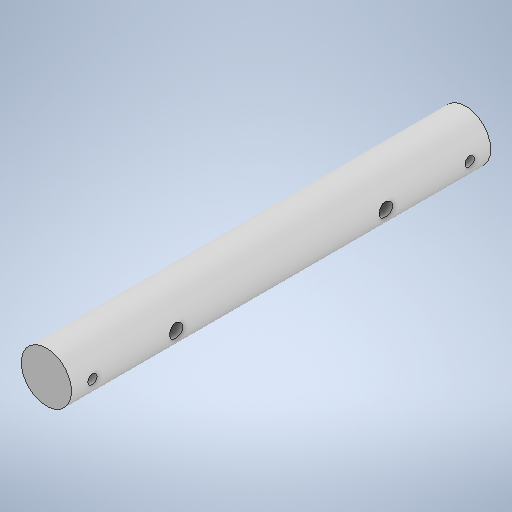
# Autodesk Inventor part: xx_jiku_kakudo
Saved by Autodesk Inventor 2025.1 (Build 291241000, 241)
## iProperties
Created: 2024-12-04
Part Number: xx_jiku_kakudo
Material: 一般
Document SubType Name: Modeling
Designer: yuki0520
Density: 1 g/cm^3
Appearance: 既定
Author: yuki0520
Autodesk Inventor part; units mm, degrees
ref_plane "YZ Plane" through (0, 0, 0) normal (1, 0, 0) x (0, 1, 0)
ref_plane "XZ Plane" through (0, 0, 0) normal (0, 1, 0) x (-1, 0, 0)
ref_plane "XY Plane" through (0, 0, 0) normal (0, 0, 1) x (1, 0, 0)
sketch "スケッチ1" plane through (0, 0, 0) normal (0, 0, 1) x (1, 0, 0)
  circle A0 centre (0, 0) radius 6
  dimension "d0" = 12
  constraints: 1 centre point, 1 coincident
  measures "d0" diameter of A0
extrude "押し出し1" add sketch "スケッチ1" along normal blind 100
sketch "スケッチ2" plane through (0, 0, 0) normal (1, 0, 0) x (0, 1, 0)
  line L0 (0, 0) -> (0, 100)
  line L1 (6, 100) -> (-6, 100) projected
  point P0 (0, 75)
  point P1 (0, 25)
  point P2 (0, 50)
  dimension "d3" = 25
  dimension "d4" = 25
  constraints: 2 end point, 2 midpoint, 2 point on line
  measures "d3" distance of point (0, 50) point (0, 25)
  measures "d4" distance of point (0, 75) point (0, 50)
hole "穴1" at (0, 0, 75) at (0, 0, 25) direction (-1, 0, 0) diameter 3.2 end through all both
sketch "スケッチ3" plane through (0, 0, 0) normal (1, 0, 0) x (0, 1, 0)
  line L0 (0, 0) -> (0, 100)
  line L1 (6, 100) -> (-6, 100) projected
  line L2 (6, 0) -> (-6, 0) projected
  point P0 (0, 95)
  point P1 (0, 5)
  dimension "d12" = 5
  dimension "d13" = 5
  constraints: 2 end point, 2 point on line, 1 midpoint
  measures "d12" distance from line of L2 point (0, 5)
  measures "d13" distance from line of L1 point (0, 95)
hole "穴2" at (0, 0, 95) at (0, 0, 5) direction (-1, 0, 0) diameter 2.2 end through all both
equation "\"d3\" = d4"
